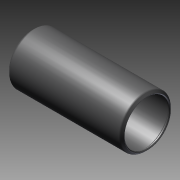
# Autodesk Inventor part: 04R-1.75550C
Saved by Autodesk Inventor 2011 SP1 (Build 150282100, 282)
## iProperties
Created: 2015-01-23
Part Number: 04R-1.75550C
Catalog Web Link: www.cadenas.de
Description: Tube-Original Line - Standard Air Cylinders
Vendor: BIMBA
Document SubType Name: Modeling
Designer: psAdmin
Manufacturer: BIMBA
Mass: 1.71231 g
Surface Area: 58.4245 cm^2
Volume: 1.71231 cm^3
Density: 1 g/cm^3
Category: PARTsolutions
Company: BIMBA
Title: 04R-1.75550C
Author: Cadenas PARTsolutions
Comments: Original Line - Standard Air Cylinders
PSOL_IDENT_0: {$CADENAS_DATA\23d-libs\bimba\bimba\bimba_imperial\bimba_full_line\original_line_cylinders\standard_
PSOL_IDENT_1: air_cylinders\tube.prj},192 {VTYP=3D},{NB=04R-1.75550C},{LINA=04R-1.75550C},{NN=Tube},{DATE=08.09.20
PSOL_IDENT_2: 14 05:03:26},{GEOMDATE=18.02.2011 00:00:00},{VERSION=},{LINEID=40},{LINESUBID=-1},{WBVAR=MNT,ACTING,
PSOL_IDENT_3: NR,L,FOURHOLES,SR}  {NB=04R-1.75550C},{LINA=04R-1.75550C},{KT=DUMMY},{PN=04R-1.75550C},{BORE=0.75000
PSOL_IDENT_4: 000},{BOREPN=04},{MNT=},{MNTALG='' , 'Front Nose' , 'BF' , 'Front Block' , 'BFT' , 'Front Trunnion'
PSOL_IDENT_5: , 'A' , 'Adjustable Stroke'},{ACTING=R},{ACTINGALG= '' , 'Single Acting' , 'R' , 'Reverse/Double Act
PSOL_IDENT_6: ing' },{NR=},{NRALG= '' , 'N/A' },{L=1.7555},{OD=0.8075},{ODN=0.8050},{ODP=0.8625},{ODB=0.8325},{ID=
PSOL_IDENT_7: 0.7615},{DV=0.00000000},{LV=0.00000000},{LV1=0.00000000},{G=0.0300},{FOURHOLES=0},{AA=0.3750},{BB=0.
PSOL_IDENT_8: 0940},{SR=C},{SRALG= 'C' , 'Carbon Steel Rod' , 'SR' , '303 Stainless Steel Rod' , '' , '303 Stainle
PSOL_IDENT_9: ss Steel Rod'}
SUPPLIER: BIMBA
ARTICLENO: 04R-1.75550C
BOMINFO: 04R-1.75550C
CREATOR: CADENAS GmbH
Autodesk Inventor part; units mm, degrees
ref_plane "YZ Plane" through (0, 0, 0) normal (1, 0, 0) x (0, 1, 0)
ref_plane "XZ Plane" through (0, 0, 0) normal (0, 1, 0) x (-1, 0, 0)
ref_plane "XY Plane" through (0, 0, 0) normal (0, 0, 1) x (1, 0, 0)
sketch "Sketch_1" plane through (0, 0, 0) normal (0, 0, 1) x (1, 0, 0)
  line L0 (44.5897, 0) -> (0, 0)
  arc A0 (-0.6395, 9.3472) -> (-0.6395, 9.1676) centre (-0.5497, 9.2574) ccw
  line L1 (-0.6395, 9.1676) -> (-0.381, 8.9091)
  line L2 (-0.381, 8.9091) -> (0, 8.9091)
  line L3 (0, 8.9091) -> (0.762, 9.671)
  line L4 (0.762, 9.671) -> (43.8277, 9.671)
  line L5 (43.8277, 9.671) -> (44.5897, 8.9091)
  line L6 (44.5897, 8.9091) -> (44.9707, 8.9091)
  line L7 (44.9707, 8.9091) -> (45.2292, 9.1676)
  arc A1 (45.2292, 9.1676) -> (45.2292, 9.3472) centre (45.1394, 9.2574) ccw
  line L8 (45.2292, 9.3472) -> (44.5443, 10.0321)
  arc A2 (44.5443, 10.0321) -> (44.0055, 10.2553) centre (44.0055, 9.4933) ccw
  line L9 (44.0055, 10.2553) -> (0.5842, 10.2553)
  arc A3 (0.5842, 10.2553) -> (0.0454, 10.0321) centre (0.5842, 9.4933) ccw
  line L10 (0.0454, 10.0321) -> (-0.6395, 9.3472)
  constraints: 22 end point, 8 point on circle, 4 centre point
revolve "Revolution1" add sketch "Sketch_1" angle 360 about axis through (44.5897, 0, 0) along (1, 0, 0)
ref_plane "cp1_XY" through (22.2949, 10.2553, 0) normal (1, 0, 0) x (0, 0, -1)
ref_plane "cp1_YZ" through (22.2949, 10.2553, 0) normal (0, 0, -1) x (0, 1, 0)
ref_plane "cp1_ZX" through (22.2949, 10.2553, 0) normal (0, 1, 0) x (1, 0, 0)
ref_plane "cp2_XY" through (22.2949, 0, -10.2553) normal (1, 0, 0) x (0, 0, -1)
ref_plane "cp2_YZ" through (22.2949, 0, -10.2553) normal (0, 0, -1) x (0, 1, 0)
ref_plane "cp2_ZX" through (22.2949, 0, -10.2553) normal (0, 1, 0) x (1, 0, 0)
ref_plane "cp3_XY" through (22.2949, -10.2553, 0) normal (1, 0, 0) x (0, 0, -1)
ref_plane "cp3_YZ" through (22.2949, -10.2553, 0) normal (0, 0, -1) x (0, 1, 0)
ref_plane "cp3_ZX" through (22.2949, -10.2553, 0) normal (0, 1, 0) x (1, 0, 0)
ref_plane "cp4_XY" through (22.2949, 0, 10.2553) normal (1, 0, 0) x (0, 0, -1)
ref_plane "cp4_YZ" through (22.2949, 0, 10.2553) normal (0, 0, -1) x (0, 1, 0)
ref_plane "cp4_ZX" through (22.2949, 0, 10.2553) normal (0, 1, 0) x (1, 0, 0)
ref_plane "tube_front_XY" through (0, 0, 0) normal (1, 0, 0) x (0, 0, -1)
ref_plane "tube_front_YZ" through (0, 0, 0) normal (0, 0, -1) x (0, 1, 0)
ref_plane "tube_front_ZX" through (0, 0, 0) normal (0, 1, 0) x (1, 0, 0)
ref_plane "tube_rear_XY" through (44.5897, 0, 0) normal (1, 0, 0) x (0, 0, -1)
ref_plane "tube_rear_YZ" through (44.5897, 0, 0) normal (0, 0, -1) x (0, 1, 0)
ref_plane "tube_rear_ZX" through (44.5897, 0, 0) normal (0, 1, 0) x (1, 0, 0)
body "Solid1"
